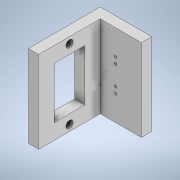
# Autodesk Inventor part: L-bracket
Saved by Autodesk Inventor 2022 (Build 260153000, 153)
## iProperties
Created: 2021-07-21
Part Number: L-bracket
Material: Generic
Document SubType Name: Modeling
Designer: WASHINGTON
Density: 1 g/cm^3
Appearance: Default
Author: WASHINGTON
Autodesk Inventor part; units mm, degrees
ref_plane "YZ Plane" through (0, 0, 0) normal (1, 0, 0) x (0, 1, 0)
ref_plane "XZ Plane" through (0, 0, 0) normal (0, 1, 0) x (-1, 0, 0)
ref_plane "XY Plane" through (0, 0, 0) normal (0, 0, 1) x (1, 0, 0)
sketch "Sketch1" plane through (0, 0, 0) normal (0, 1, 0) x (-1, 0, 0)
  line L0 (0, 0) -> (50, 0)
  line L1 (50, 0) -> (50, 3.3201)
  line L2 (40, 10) -> (0, 10)
  line L3 (0, 10) -> (0, 0)
  line L4 (50, 70) -> (40, 70)
  line L5 (40, 70) -> (40, 10)
  line L6 (50, 3.3201) -> (50, 70)
  dimension "d0" = 50
  dimension "d1" = 70
  dimension "d2" = 10
  dimension "d3" = 10
  constraints: 14 end point, 3 parallel, 2 horizontal, 2 perpendicular, 1 point on line
  measures "d0" distance of L0.start L0.end
  measures "d1" distance of L4.start L0.end
  measures "d2" distance of L4.start L4.end
  measures "d3" distance of L2.end L0.start
extrude "Extrusion1" add sketch "Sketch1" along normal mid plane 80
sketch "Sketch2" plane through (-40, -40, 10) normal (1, 0, 0) x (0, 0, -1)
  line L0 (-45, 65) -> (-15, 65)
  line L1 (-15, 65) -> (-15, 15)
  line L2 (-15, 15) -> (-45, 15)
  line L3 (-45, 15) -> (-45, 65)
  line L4 (-60, 80) -> (0, 80) projected
  line L5 (-60, 0) -> (-60, 80) projected
  point P0 (10, 40)
  dimension "d6" = 30
  dimension "d7" = 50
  dimension "d8" = 15
  dimension "d9" = 15
  constraints: 8 end point, 2 parallel, 1 horizontal, 1 perpendicular
  measures "d6" distance of L0.start L0.end
  measures "d7" distance of L2.end L0.start
  measures "d8" distance between parallel lines of L4 L0
  measures "d9" distance between parallel lines of L5 L3
extrude "Extrusion2" cut sketch "Sketch2" against normal through all
sketch "Sketch3" plane through (-40, -40, 10) normal (1, 0, 0) x (0, 0, -1)
  circle A0 centre (-30, 74) radius 3.5
  circle A1 centre (-30, 6) radius 3.5
  line L0 (-60, 0) -> (-60, 80) projected
  line L1 (-60, 80) -> (0, 80) projected
  point P0 (10, 40)
  dimension "d12" = 7
  dimension "d13" = 7
  dimension "d14" = 30
  dimension "d15" = 68
  dimension "d16" = 6
  dimension "d17" = 30
  constraints: 2 centre point
  measures "d12" diameter of A1
  measures "d13" diameter of A0
  measures "d14" distance from line of A0.centre L0
  measures "d15" distance of A1.centre A0.centre
  measures "d16" distance from line of L1 A0.centre
  measures "d17" distance from line of L0 A1.centre
extrude "Extrusion3" cut sketch "Sketch3" against normal through all
sketch "Sketch4" plane through (0, 40, 0) normal (0, 0, -1) x (-1, 0, 0)
  circle A0 centre (25, -24.5) radius 1.25
  circle A1 centre (25, -30.5) radius 1.25
  circle A2 centre (25, -49.5) radius 1.25
  circle A3 centre (25, -55.5) radius 1.25
  line L0 (0, -80) -> (0, 0) projected
  line L1 (50, -80) -> (0, -80) projected
  point P0 (0, -40)
  dimension "d20" = 2.5
  dimension "d21" = 31
  dimension "d22" = 19
  dimension "d23" = 6
  dimension "d24" = 6
  dimension "d25" = 25
  dimension "d26" = 24.5
  dimension "d32" = 2.5
  dimension "d33" = 2.5
  dimension "d34" = 2.5
  dimension "d35" = 55.5
  dimension "d36" = 49.5
  constraints: 4 centre point
  measures "d20" diameter of A0
  measures "d21" distance of A3.centre A0.centre
  measures "d22" distance of A2.centre A1.centre
  measures "d23" distance of A0.centre A1.centre
  measures "d24" distance of A3.centre A2.centre
  measures "d25" distance from line of L0 A0.centre
  measures "d26" distance from line of L1 A3.centre
  measures "d32" diameter of A1
  measures "d33" diameter of A2
  measures "d34" diameter of A3
  measures "d35" distance from line of A0.centre L1
  measures "d36" distance from line of A1.centre L1
extrude "Extrusion4" cut sketch "Sketch4" against normal through all
body "Solid1"
